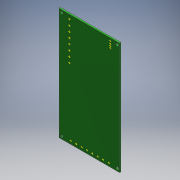
# Autodesk Inventor part: powerDistributionPCB
Saved by Autodesk Inventor 2016 (Build 200138000, 138)
## iProperties
Created: 2015-12-24
Part Number: powerDistributionPCB
Material: GFRP
Document SubType Name: Modeling
Designer: Artur
Density: 1.75 g/cm^3
Appearance: Smooth - Light Gray
Mass: 27.3822 g
Surface Area: 204.737 cm^2
Volume: 15.647 cm^3
Author: Artur
Autodesk Inventor part; units mm, degrees
ref_plane "YZ Plane" through (0, 0, 0) normal (1, 0, 0) x (0, 1, 0)
ref_plane "XZ Plane" through (0, 0, 0) normal (0, 1, 0) x (-1, 0, 0)
ref_plane "XY Plane" through (0, 0, 0) normal (0, 0, 1) x (1, 0, 0)
sketch "Sketch1" plane through (0, 0, 0) normal (0, 1, 0) x (-1, 0, 0)
  line L0 (0, 0) -> (0, -135)
  line L1 (0, -135) -> (73.0002, -135)
  line L2 (73.0002, -135) -> (73.0002, 0)
  circle A0 centre (3, -3) radius 1.75
  line L3 (73.0002, 0) -> (0, 0)
  circle A1 centre (70.0002, -3) radius 1.75
  circle A2 centre (70.0002, -132) radius 1.75
  circle A3 centre (3, -132) radius 1.75
  circle A4 centre (13, -131) radius 0.75
  circle A5 centre (19.5, -131) radius 0.75
  circle A6 centre (26, -131) radius 0.75
  circle A7 centre (32.5, -131) radius 0.75
  circle A8 centre (39, -131) radius 0.75
  circle A9 centre (45.5, -131) radius 0.75
  circle A10 centre (52, -131) radius 0.75
  circle A11 centre (58.5, -131) radius 0.75
  circle A12 centre (11, -3) radius 0.55
  circle A13 centre (11, -5.54) radius 0.55
  circle A14 centre (11, -8.08) radius 0.55
  circle A15 centre (11, -10.62) radius 0.55
  circle A16 centre (60.0002, -5) radius 0.75
  circle A17 centre (60.0002, -11.5) radius 0.75
  circle A18 centre (60.0002, -18) radius 0.75
  circle A19 centre (60.0002, -24.5) radius 0.75
  circle A20 centre (60.0002, -31) radius 0.75
  circle A21 centre (60.0002, -37.5) radius 0.75
  circle A22 centre (60.0002, -44) radius 0.75
  circle A23 centre (60.0002, -50.5) radius 0.75
  line L4 (47, -21) -> (26, -21) construction
  line L5 (44, -53) -> (23, -53) construction
  line L6 (47, -85) -> (26, -85) construction
  line L7 (50, -115) -> (29, -115) construction
  line L8 (47, -21) -> (47, -11.5) construction
  line L9 (26, -21) -> (26, -11.5) construction
  line L10 (44, -53) -> (44, -43.5) construction
  line L11 (23, -53) -> (23, -43.5) construction
  line L12 (26, -85) -> (26, -75.5) construction
  line L13 (47, -85) -> (47, -75.5) construction
  line L14 (50, -115) -> (50, -105.5) construction
  line L15 (29, -115) -> (29, -105.5) construction
  circle A24 centre (29, -105.5) radius 0.45
  circle A25 centre (50, -105.5) radius 0.45
  circle A26 centre (47, -75.5) radius 0.45
  circle A27 centre (26, -75.5) radius 0.45
  circle A28 centre (44, -43.5) radius 0.45
  circle A29 centre (23, -43.5) radius 0.45
  circle A30 centre (26, -11.5) radius 0.45
  circle A31 centre (47, -11.5) radius 0.45
  dimension "d42" = 3.5
  dimension "d52" = 3
  dimension "d53" = 3
  dimension "d54" = 135
  dimension "d55" = 73.0002
  dimension "d56" = 3.5
  dimension "d57" = 3.5
  dimension "d58" = 3.5
  dimension "d59" = 3
  dimension "d60" = 3
  dimension "d61" = 3
  dimension "d62" = 3
  dimension "d63" = 3
  dimension "d64" = 3
  dimension "d65" = 1.5
  dimension "d66" = 4
  dimension "d67" = 13
  dimension "d70" = 6.5
  dimension "d75" = 1.1
  dimension "d76" = 3
  dimension "d77" = 11
  dimension "d80" = 2.54
  dimension "d85" = 1.5
  dimension "d86" = 13
  dimension "d87" = 5
  dimension "d90" = 6.5
  dimension "d95" = 21
  dimension "d96" = 21
  dimension "d97" = 21
  dimension "d98" = 21
  dimension "d99" = 26
  dimension "d100" = 114
  dimension "d101" = 23
  dimension "d102" = 82
  dimension "d103" = 26
  dimension "d104" = 50
  dimension "d105" = 29
  dimension "d106" = 20
  dimension "d115" = 0.9
  dimension "d128" = 0.9
  dimension "d141" = 0.9
  dimension "d154" = 0.9
  dimension "d167" = 0.9
  dimension "d180" = 0.9
  dimension "d193" = 0.9
  dimension "d206" = 0.9
  dimension "d209" = 9.5
  dimension "d210" = 9.5
  dimension "d211" = 9.5
  dimension "d212" = 9.5
  dimension "d213" = 9.5
  dimension "d214" = 9.5
  dimension "d215" = 9.5
  dimension "d216" = 9.5
  constraints: 32 centre point, 32 end point, 10 coincident, 7 horizontal, 6 parallel, 6 vertical, 34 other
  measures "d42" diameter of A0
  measures "d52" distance from line of L0 point (3, -3)
  measures "d53" distance from line of L3 point (3, -3)
  measures "d54" distance of L0.start L0.end
  measures "d55" distance of L2.end L0.start
  measures "d56" diameter of A1
  measures "d57" diameter of A2
  measures "d58" diameter of A3
  measures "d59" distance from line of L3 A1.centre
  measures "d60" distance from line of L2 A1.centre
  measures "d61" distance from line of L2 A2.centre
  measures "d62" distance from line of L1 A2.centre
  measures "d63" distance from line of L1 A3.centre
  measures "d64" distance from line of L0 A3.centre
  measures "d65" diameter of A4
  measures "d66" distance from line of L1 A4.centre
  measures "d67" distance from line of L0 A4.centre
  measures "d70" distance of A4.centre A5.centre
  measures "d75" diameter of A12
  measures "d76" distance from line of L3 A12.centre
  measures "d77" distance from line of L0 A12.centre
  measures "d80" distance of A12.centre A13.centre
  measures "d85" diameter of A16
  measures "d86" distance from line of L2 A16.centre
  measures "d87" distance from line of L3 A16.centre
  measures "d90" distance of A16.centre A17.centre
  measures "d95" distance of L7.start L7.end
  measures "d96" distance of L6.start L6.end
  measures "d97" distance of L5.start L5.end
  measures "d98" distance of L4.start L4.end
  measures "d99" distance from line of L0 L4.end
  measures "d100" distance from line of L1 L4.end
  measures "d101" distance from line of L0 L5.end
  measures "d102" distance from line of L1 L5.end
  measures "d103" distance from line of L0 L6.end
  measures "d104" distance from line of L1 L6.end
  measures "d105" distance from line of L0 L7.end
  measures "d106" distance from line of L1 L7.end
  measures "d115" diameter of A24
  measures "d128" diameter of A25
  measures "d141" diameter of A26
  measures "d154" diameter of A27
  measures "d167" diameter of A28
  measures "d180" diameter of A29
  measures "d193" diameter of A30
  measures "d206" diameter of A31
  measures "d209" distance of L4.end L9.end
  measures "d210" distance of L4.start L8.end
  measures "d211" distance of L5.start L10.end
  measures "d212" distance of L5.end L11.end
  measures "d213" distance of L6.start L13.end
  measures "d214" distance of L6.end L12.end
  measures "d215" distance of L7.start L14.end
  measures "d216" distance of L7.end L15.end
extrude "Extrusion1" add sketch "Sketch1" along normal blind 1.6
sketch "Sketch2" plane through (0, 0, 0) normal (0, -1, 0) x (1, 0, 0)
  circle A0 centre (-60.0002, -5) radius 0.75 construction
  circle A1 centre (-60.0002, -11.5) radius 0.75 construction
  circle A2 centre (-60.0002, -18) radius 0.75 construction
  circle A3 centre (-60.0002, -24.5) radius 0.75 construction
  circle A4 centre (-60.0002, -31) radius 0.75 construction
  circle A5 centre (-11, -3) radius 0.55 construction
  circle A6 centre (-11, -5.54) radius 0.55 construction
  circle A7 centre (-11, -8.08) radius 0.55 construction
  circle A8 centre (-11, -10.62) radius 0.55 construction
  circle A9 centre (-60.0002, -37.5) radius 0.75 construction
  circle A10 centre (-60.0002, -44) radius 0.75 construction
  circle A11 centre (-60.0002, -50.5) radius 0.75 construction
  circle A12 centre (-58.5, -131) radius 0.75 construction
  circle A13 centre (-52, -131) radius 0.75 construction
  circle A14 centre (-45.5, -131) radius 0.75 construction
  circle A15 centre (-39, -131) radius 0.75 construction
  circle A16 centre (-26, -131) radius 0.75 construction
  circle A17 centre (-19.5, -131) radius 0.75 construction
  circle A18 centre (-13, -131) radius 0.75 construction
  circle A19 centre (-32.5, -131) radius 0.75 construction
  circle A20 centre (-60.0002, -31) radius 0.75 construction
  circle A21 centre (-60.0002, -24.5) radius 0.75 construction
  circle A22 centre (-60.0002, -11.5) radius 0.75 projected
  point P0 (0, 0)
  constraints: 20 coincident
body "Solid1"
